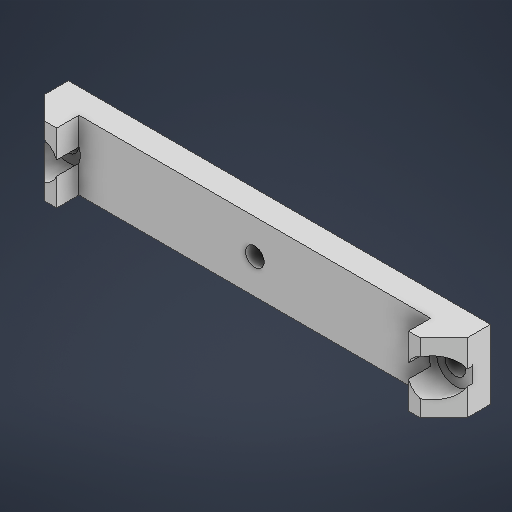
# Autodesk Inventor part: GA_FixaBase
Saved by Autodesk Inventor 2025.2 (Build 292293000, 293)
## iProperties
Created: 2025-07-02
Part Number: GA_FixaBase
Material: Generic
Document SubType Name: Modeling
Designer: Tiago
Density: 1 g/cm^3
Appearance: Default
Author: Tiago
Autodesk Inventor part; units mm, degrees
ref_plane "YZ Plane" through (0, 0, 0) normal (1, 0, 0) x (0, 1, 0)
ref_plane "XZ Plane" through (0, 0, 0) normal (0, 1, 0) x (-1, 0, 0)
ref_plane "XY Plane" through (0, 0, 0) normal (0, 0, 1) x (1, 0, 0)
sketch "Sketch1" plane through (0, 0, 0) normal (0, 0, 1) x (1, 0, 0)
  line L0 (-36, 5.9) -> (36, 5.9)
  line L1 (36, 5.9) -> (36, -5.9)
  line L2 (36, -5.9) -> (-36, -5.9)
  line L3 (-36, -5.9) -> (-36, 5.9)
  line L4 (-30, 5.9) -> (-30, -5.9)
  line L5 (30, 5.9) -> (30, -5.9)
  point P0 (0, 0)
  point P1 (0, 5.9)
  point P2 (-36, 0)
  dimension "d0" = 11.8
  dimension "d1" = 72
  dimension "d2" = 6
  dimension "d3" = 6
  constraints: 12 end point, 4 point on line, 3 perpendicular, 2 midpoint, 2 parallel, 1 horizontal, 1 horizontal alignment, 1 vertical alignment
  measures "d0" distance of L0.end L1.end
  measures "d1" distance of L0.start L0.end
  measures "d2" distance between parallel lines of L1 L5
  measures "d3" distance between parallel lines of L3 L4
extrude "Extrusion1" add sketch "Sketch1" along normal blind 4.2
extrude "Extrusion2" add sketch "Sketch1" along normal blind 8 contours L0 L4 L2 L3 | L0 L1 L2 L5
sketch "Sketch2" plane through (0, 0, 8) normal (0, 0, 1) x (1, 0, 0)
  circle A0 centre (-33.022, 0) radius 3.25
  circle A1 centre (-33.022, 0) radius 1.75
  circle A2 centre (0, 0) radius 1.6
  line L0 (0, 3.25) -> (0, 0) construction
  circle A3 centre (33.022, 0) radius 3.25
  circle A4 centre (33.022, 0) radius 1.75
  dimension "d9" = 6.5
  dimension "d10" = 33.022
  dimension "d11" = 3.5
  dimension "d12" = 3.2
  constraints: 5 centre point, 3 coincident, 2 end point, 2 symmetric about line, 1 horizontal alignment, 1 vertical, 2 other
  measures "d9" diameter of A0
  measures "d10" distance of point (0, 0) A0.centre
  measures "d11" diameter of A1
  measures "d12" diameter of A2
extrude "Extrusion3" cut sketch "Sketch2" against normal up to surface (8 mm away) contours A1 | A2 | A4
chamfer "Chamfer1" distance 4 angle 45 2 edges at (-36, 0, 8) (36, 0, 8)
extrude "Extrusion4" cut sketch "Sketch2" against normal blind 5 contours A0 | A3
body "Solid1"
